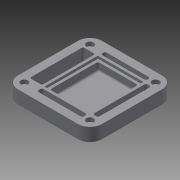
# Autodesk Inventor part: new IC holder
Saved by Autodesk Inventor 2015 (Build 190159000, 159)
## iProperties
Created: 2014-12-11
Part Number: new IC holder
Material: Generic
Document SubType Name: Modeling
Designer: Purple
Density: 1 g/cm^3
Appearance: Default
Author: Purple
Autodesk Inventor part; units mm, degrees
ref_plane "YZ Plane" through (0, 0, 0) normal (1, 0, 0) x (0, 1, 0)
ref_plane "XZ Plane" through (0, 0, 0) normal (0, 1, 0) x (-1, 0, 0)
sketch "Sketch1" plane through (0, 0, 0) normal (0, 1, 0) x (-1, 0, 0)
  line L0 (30, 30) -> (-30, 30)
  line L1 (-30, 30) -> (-30, -30)
  line L2 (-30, -30) -> (30, -30)
  line L3 (30, -30) -> (30, 30)
  line L4 (30, 30) -> (-30, -30) construction
  line L5 (-30, 30) -> (30, -30) construction
  point P0 (0, 0)
  dimension "d0" = 60
  dimension "d1" = 60
  constraints: 12 end point, 2 midpoint, 2 parallel, 1 horizontal, 1 perpendicular
  measures "d0" distance of L2.end L1.end
  measures "d1" distance of L0.end L1.end
extrude "Extrusion1" add sketch "Sketch1" along normal blind 10
fillet "Fillet1" radius 7 4 edges at (30, 5, 30) (30, 5, -30) (-30, 5, 30) (-30, 5, -30)
sketch "Sketch2" plane through (0, 10, 0) normal (0, 1, 0) x (1, 0, 0)
  line L0 (-30, 30) -> (30, 30)
  line L1 (30, 30) -> (30, -30)
  line L2 (30, -30) -> (-30, -30)
  line L3 (-30, -30) -> (-30, 30)
  line L4 (-30, 30) -> (30, -30) construction
  line L5 (30, 30) -> (-30, -30) construction
  line L6 (25, -25) -> (25, 25)
  line L7 (25, 25) -> (-25, 25)
  line L8 (-25, 25) -> (-25, -25)
  line L9 (-25, -25) -> (25, -25)
  circle A0 centre (25, -25) radius 2.75
  circle A1 centre (-25, -25) radius 2.75
  circle A2 centre (25, 25) radius 2.75
  circle A3 centre (-25, 25) radius 2.75
  point P0 (0, 0)
  dimension "d5" = 5
  dimension "d6" = 5.5
  dimension "d7" = 5.5
  dimension "d8" = 5.5
  dimension "d9" = 5.5
  constraints: 20 end point, 4 centre point, 4 coincident, 4 parallel, 2 midpoint, 2 perpendicular, 1 horizontal, 3 other
  measures "d5" distance between parallel lines of L1 L6
  measures "d6" diameter of A0
  measures "d7" diameter of A1
  measures "d8" diameter of A2
  measures "d9" diameter of A3
extrude "Extrusion2" cut sketch "Sketch2" against normal blind 3 contours L9 A0 L6 | L6 A0 L9 | A2 L7 L6 | L6 L7 A2 | A1 L8 L9 | L9 L8 A1 | A3 L8 L7 | L7 L8 A3
sketch "Sketch3" plane through (0, 10, 0) normal (0, 1, 0) x (1, 0, 0)
  line L0 (-30, 30) -> (30, 30)
  line L1 (30, 30) -> (30, -30)
  line L2 (30, -30) -> (-30, -30)
  line L3 (-30, -30) -> (-30, 30)
  line L4 (-30, 30) -> (30, -30) construction
  line L5 (30, 30) -> (-30, -30) construction
  line L6 (20, -20) -> (20, 20.65)
  line L7 (-20, -20) -> (20, -20)
  line L8 (18, 18.65) -> (18, -18)
  line L9 (-20, 20.65) -> (20.65, 20.65)
  line L10 (18, 18.65) -> (18.65, 18.65)
  line L11 (-12.6, -18) -> (-12.6, 18.65)
  line L12 (-14.6, -20) -> (-14.6, 20.65)
  line L13 (18, 18.65) -> (-12.6, 18.65)
  line L14 (18, -18) -> (-12.6, -18)
  line L15 (-26, 20.65) -> (-20, 20.65)
  line L16 (-26, 20.65) -> (-26, -20)
  line L17 (-26, -20) -> (-20, -20)
  point P0 (0, 0)
  point P1 (-12.6, -20)
  dimension "d12" = 60
  dimension "d13" = 60
  dimension "d14" = 10
  dimension "d16" = 34.6
  dimension "d17" = 2
  dimension "d18" = 40.65
  dimension "d22" = 4
  dimension "d23" = 4
  constraints: 36 end point, 5 point on line, 4 perpendicular, 2 horizontal, 2 midpoint, 2 parallel, 1 collinear
  measures "d12" distance of L1.end L2.end
  measures "d13" distance of L0.end L1.end
  measures "d14" distance between parallel lines of L1 L6
  measures "d16" distance of L6.start L12.start
  measures "d17" distance of L12.start point (-12.6, -20)
  measures "d18" distance of L6.end L6.start
  measures "d22" distance from line of L3 L15.start
  measures "d23" distance from line of L3 L16.end
extrude "Extrusion3" cut sketch "Sketch3" against normal blind 2 contours L7 L12 L9 L6
sketch "Sketch4" plane through (0, 10, 0) normal (0, 1, 0) x (1, 0, 0)
  line L0 (-12.6, 18.65) -> (18, 18.65)
  line L1 (18, 18.65) -> (18, -18)
  line L2 (18, -18) -> (-12.6, -18)
  line L3 (-12.6, -18) -> (-12.6, 18.65)
  point P0 (0, 0)
  constraints: 8 end point, 2 parallel, 1 horizontal, 1 perpendicular
extrude "Extrusion4" cut sketch "Sketch4" against normal blind 8
sketch "Sketch5" plane through (0, 10, 0) normal (0, 1, 0) x (1, 0, 0)
  line L0 (20, -20) -> (-14.6, -20)
  line L1 (-14.6, -20) -> (-14.6, 20.65)
  line L2 (-30, 23) -> (-30, -23) projected
  line L3 (-23, -30) -> (23, -30) projected
  line L4 (30, -23) -> (30, 23) projected
  line L5 (-26, 20.65) -> (-14.6, 20.65)
  line L6 (-26, -20) -> (-14.6, -20)
  line L7 (-26, 20.65) -> (-26, -20)
  line L8 (-14.6, -26) -> (-14.6, -20)
  line L9 (-14.6, -20) -> (-14.6, -26)
  line L10 (20, -26) -> (-14.6, -26)
  line L11 (20, -20) -> (20, -26)
  line L12 (26, -20) -> (20, -20)
  line L13 (26, 20.65) -> (20, 20.65)
  line L14 (30, -23) -> (30, 23) projected
  line L15 (26, 20.65) -> (26, -20)
  line L16 (23, 30) -> (-23, 30) projected
  line L17 (-14.6, 26) -> (-14.6, 20.65)
  line L18 (-14.6, 26) -> (20, 26)
  line L19 (20, 26) -> (20, 20.65)
  line L20 (-16.6, -20) -> (-16.6, 20.65)
  line L21 (20, -22) -> (-14.6, -22)
  line L22 (22, 20.65) -> (22, -20)
  line L23 (-14.6, 22.65) -> (18.1816, 22.65)
  line L24 (18.1816, 22.65) -> (20, 22.65)
  point P0 (0, 0)
  dimension "d28" = 4
  dimension "d29" = 4
  dimension "d30" = 4
  dimension "d31" = 4
  dimension "d32" = 4
  dimension "d33" = 4
  dimension "d36" = 4
  dimension "d37" = 4
  dimension "d38" = 2
  dimension "d39" = 2
  constraints: 40 end point, 8 point on line, 6 perpendicular, 4 equal length, 2 horizontal, 1 vertical
  measures "d28" distance from line of L2 L5.start
  measures "d29" distance from line of L2 L6.start
  measures "d30" distance from line of L3 L8.start
  measures "d31" distance from line of L3 L10.start
  measures "d32" distance from line of L4 L12.start
  measures "d33" distance from line of L4 L13.start
  measures "d36" distance from line of L17.start L16
  measures "d37" distance from line of L18.end L16
  measures "d38" distance between parallel lines of L1 L20
  measures "d39" distance between parallel lines of L0 L21
extrude "Extrusion5" cut sketch "Sketch5" against normal through all contours L11 L10 L8 L21 | L22 L13 L15 L12 | L6 L7 L5 L20 | L17 L18 L19 L24 L23
fillet "Fillet2" radius 1.5 24 edges at (-16.6, 5, -20.65) (20, 5, -26) (26, 5, -20.65) (20, 5, 22) (-14.6, 5, -26) (-26, 5, -20.65) (22, 5, -20.65) (-14.6, 5, 22) (-26, 5, 20) (-14.6, 5, -22.65) (-14.6, 5, 26) (-16.6, 5, 20) (20, 5, 26) (26, 5, 20) (18, 2, -0.325) (2.7, 2, 18) (-12.6, 2, -0.325) (2.7, 2, -18.65) (-12.6, 5, -18.65) (18, 5, -18.65) (18, 5, 18) (-12.6, 5, 18) (22, 5, 20) (20, 5, -22.65)
sketch "Sketch6" plane through (-12.6, 3.5, 16.5) normal (1, 0, 0) x (0, 0, -1)
  point P0 (16.5, -3.5)
ref_plane "Work Plane1" through (0, 5, 0) normal (0, 1, 0) x (1, 0, 0)
mirror "Mirror1" about plane through (0, 5, 0) normal (0, 1, 0) of "Extrusion2"
sketch "Sketch7" plane through (0, 10, 0) normal (0, 1, 0) x (1, 0, 0)
  line L0 (-23, 30) -> (23, 30)
  line L1 (30, 23) -> (30, -23)
  line L2 (23, -30) -> (-23, -30)
  line L3 (-30, -23) -> (-30, 23)
  line L4 (-30, 30) -> (30, -30) construction
  line L5 (30, 30) -> (-30, -30) construction
  arc A0 (30, 23) -> (23, 30) centre (23, 23) ccw
  arc A1 (-23, 30) -> (-30, 23) centre (-23, 23) ccw
  arc A2 (-30, -23) -> (-23, -30) centre (-23, -23) ccw
  arc A3 (23, -30) -> (30, -23) centre (23, -23) ccw
  line L6 (32, -23) -> (32, 23)
  arc A4 (32, 23) -> (23, 32) centre (23, 23) ccw
  line L7 (23, 32) -> (-23, 32)
  arc A5 (-23, 32) -> (-32, 23) centre (-23, 23) ccw
  line L8 (-32, 23) -> (-32, -23)
  arc A6 (-32, -23) -> (-23, -32) centre (-23, -23) ccw
  line L9 (-23, -32) -> (23, -32)
  arc A7 (23, -32) -> (32, -23) centre (23, -23) ccw
  point P0 (0, 0)
  dimension "d45" = 60
  dimension "d46" = 60
  dimension "d47" = 7
  dimension "d48" = 2
  constraints: 20 end point, 16 point on circle, 8 centre point, 8 point on line, 8 tangent, 4 parallel, 3 equal radius, 2 midpoint, 2 perpendicular, 1 horizontal, 7 other
  measures "d45" distance of L4.end L5.end
  measures "d46" distance of L5.start L4.end
  measures "d47" radius of A0
  measures "d48" distance between parallel lines of L1 L6
extrude "Extrusion6" add sketch "Sketch7" against normal blind 10
body "Solid1"
